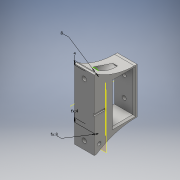
# Autodesk Inventor part: espaceur_20mm_v4
Saved by Autodesk Inventor 2016 (Build 200138000, 138)
## iProperties
Created: 2018-02-21
Part Number: espaceur_20mm_v4
Material: Generic
Document SubType Name: Modeling
Designer: mbouhier
Density: 1 g/cm^3
Appearance: Default
Author: mbouhier
Autodesk Inventor part; units mm, degrees
note: some values were not read from the file. Chosen so that the rebuilt part matches the saved one: sketch regions of "Extrusion1"; direction of "Hole1".
ref_plane "YZ Plane" through (0, 0, 0) normal (1, 0, 0) x (0, 1, 0)
ref_plane "XZ Plane" through (0, 0, 0) normal (0, 1, 0) x (-1, 0, 0)
ref_plane "XY Plane" through (0, 0, 0) normal (0, 0, 1) x (1, 0, 0)
sketch "Sketch1" plane through (0, 0, 0) normal (1, 0, 0) x (0, 1, 0)
  line L0 (0, 0) -> (0, -35.25)
  line L1 (0, -35.25) -> (2, -35.25)
  line L2 (19.75, 20.25) -> (40.25, 20.25)
  line L3 (40.25, 20.25) -> (40.25, -20.25)
  line L4 (40.25, -20.25) -> (19.75, -20.25)
  line L5 (19.75, -20.25) -> (19.75, 20.25)
  line L6 (19.75, 20.25) -> (40.25, -20.25) construction
  line L7 (40.25, 20.25) -> (19.75, -20.25) construction
  line L8 (16.75, 23) -> (43.25, 23)
  line L9 (43.25, 23) -> (43.25, -23)
  line L10 (43.25, -23) -> (16.75, -23)
  line L11 (16.75, -23) -> (16.75, 23)
  line L12 (16.75, 23) -> (43.25, -23) construction
  line L13 (43.25, 23) -> (16.75, -23) construction
  line L14 (0, 0) -> (0, 35.25)
  line L15 (0, 35.25) -> (2, 35.25)
  arc A0 (2, 35.25) -> (43.25, 23) centre (41.9161, 94.0847) ccw
  arc A1 (43.25, -23) -> (2, -35.25) centre (42.6775, -96.6486) ccw
  line L16 (-8.65, 0) -> (51.9, 0) projected
  point P0 (20, 0)
  point P1 (40.1, 0)
  point P2 (30, 0)
  point P3 (30, 23)
  point P4 (30.2, -23)
  point P5 (30, 0)
  dimension "d0" = 35.25
  dimension "d1" = 2
  dimension "d2" = 20
  dimension "d4" = 20.5
  dimension "d5" = 40.5
  dimension "d6" = 46
  dimension "d7" = 26.5
  dimension "d8" = 35.25
  constraints: 32 end point, 6 midpoint, 4 parallel, 4 point on circle, 3 horizontal, 3 perpendicular, 2 centre point, 2 point on line, 2 vertical
  measures "d0" distance of L0.start L0.end
  measures "d1" distance of L0.end L1.end
  measures "d2" distance of point (20, 0) L0.start
  measures "d4" distance of L3.end L4.end
  measures "d5" distance of L2.end L3.end
  measures "d6" distance of L8.end L9.end
  measures "d7" distance of L8.start L8.end
  measures "d8" distance of L0.start L14.end
extrude "Extrusion1" add sketch "Sketch1" along normal blind 20 contours L10 L11 L16 L5 L4 L3 L9 | L16 L11 L10 A1 L1 L0 | L14 L15 A0 L8 L11 L16 | L11 L8 A0 L9 L16 L3 L2 L5 | L8 A0
sketch "Sketch2" plane through (0, 43.25, 23) normal (0, 1, 0) x (1, 0, 0)
  line L0 (0, 46) -> (0, 0) projected
  line L1 (0, 0) -> (20, 0) projected
  line L2 (20, 46) -> (20, 0) projected
  line L3 (0, 46) -> (20, 46) projected
  line L4 (0, 2.75) -> (20, 2.75) projected
  line L5 (0, 2.75) -> (20, 2.75) projected
  point P0 (0, 23)
  point P1 (10, 12.8)
  point P2 (10, 32.8)
  dimension "d33" = 20
  dimension "d34" = 10.05
  measures "d33" distance of point (10, 32.8) point (10, 12.8)
  measures "d34" distance from line of point (10, 12.8) L4
hole "Hole1" at (10, 43.25, 10.2) at (10, 43.25, -9.8) direction (0, -1, 0) diameter 4 end up to surface
ref_plane "Work Plane1" through (0, 11, -35.25) normal (0, -1, 0) x (1, 0, 0)
sketch "Sketch3" plane through (0, 11, -35.25) normal (0, -1, 0) x (1, 0, 0)
  circle A0 centre (10, 45.45) radius 2 projected
  line L0 (0, 12.25) -> (0, 58.25) projected
  line L1 (0, 58.25) -> (20, 58.25) projected
  line L2 (20, 12.25) -> (20, 58.25) projected
  line L3 (0, 12.25) -> (20, 12.25) projected
  line L4 (0, 55.5) -> (0, 15) projected
  line L5 (0, 55.5) -> (20, 55.5) projected
  line L6 (20, 15) -> (20, 55.5) projected
  line L7 (0, 15) -> (20, 15) projected
  circle A1 centre (10, 62.25) radius 4
  circle A2 centre (10, 8.25) radius 4
  point P0 (0, 35.25)
  dimension "d19" = 4
  dimension "d20" = 4
  dimension "d30" = 8
  dimension "d31" = 8
  constraints: 2 centre point, 2 coincident
  measures "d19" distance from line of point (10, 62.25) L1
  measures "d20" distance from line of L3 point (10, 8.25)
  measures "d30" diameter of A1
  measures "d31" diameter of A2
extrude "Extrusion2" cut sketch "Sketch3" against normal blind 20 contours A1 | A2
hole "Hole2" at (10, 11, 27) at (10, 11, -27) direction (0, -1, 0) diameter 4.5 end through all
chamfer "Chamfer1" distance 1.5 angle 45 4 edges at (20, 40.25, 0) (20, 30, 20.25) (20, 19.75, 0) (20, 30, -20.25)
sketch "Sketch4" plane through (20, 0, 0) normal (1, 0, 0) x (0, 0, -1)
  line L0 (0, -8.65) -> (0, 51.9) projected
  line L1 (-35.25, 0) -> (35.25, 0) projected
  line L2 (0, 0) -> (-1, 0)
  line L3 (-1, 0) -> (-1, 11)
  line L4 (-1, 11) -> (0, 11)
  line L5 (0, 11) -> (0, 0)
  line L6 (0, 11) -> (1, 11)
  line L7 (1, 11) -> (1, 0)
  line L8 (1, 0) -> (0, 0)
  line L9 (0, 0) -> (0, 11)
  dimension "d51" = 1
  dimension "d52" = 1
  constraints: 16 end point, 4 parallel, 2 horizontal, 2 perpendicular, 1 point on line
  measures "d51" distance between parallel lines of L0 L3
  measures "d52" distance between parallel lines of L7 L0
extrude "Extrusion3" cut sketch "Sketch4" against normal blind 1
sketch "Sketch5" plane through (20, 0, 0) normal (1, 0, 0) x (0, 0, -1)
  line L0 (0, 0) -> (35.25, 0) projected
  line L1 (35.25, 0) -> (35.25, 2) projected
  point P0 (27.25, 5)
  dimension "d42" = 5
  dimension "d43" = 8
  measures "d42" distance from line of point (27.25, 5) L0
  measures "d43" distance from line of point (27.25, 5) L1
hole "Hole3" at (20, 5, -27.25) direction (-1, 0, 0) diameter 3.5 depth 5
equation "\"d8\" = d0"
equation "\"d20\" = d19"
equation "\"d31\" = d30"
equation "\"d52\" = d51"
body "Solid1"
